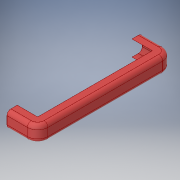
# Autodesk Inventor part: Bumper Fabric
Saved by Autodesk Inventor 2019.4 (Build 234330000, 330)
## iProperties
Created: 2020-01-22
Part Number: Bumper Fabric
Material: Fabric
Document SubType Name: Modeling
Designer: admin
Density: 0.9 g/cm^3
Appearance: Smooth - Red
Author: admin
Autodesk Inventor part; units mm, degrees
ref_plane "YZ Plane" through (0, 0, 0) normal (1, 0, 0) x (0, 1, 0)
ref_plane "XZ Plane" through (0, 0, 0) normal (0, 1, 0) x (-1, 0, 0)
ref_plane "XY Plane" through (0, 0, 0) normal (0, 0, 1) x (1, 0, 0)
sketch "Sketch1" plane through (0, 0, 0) normal (1, 0, 0) x (0, 1, 0)
  line L0 (0, 0) -> (0, 51.5)
  arc A0 (0, 51.5) -> (-31.5, 83) centre (-31.5, 51.5) ccw
  line L1 (-31.5, 83) -> (-95.5, 83)
  arc A1 (-95.5, 83) -> (-127, 51.5) centre (-95.5, 51.5) ccw
  line L2 (-127, 51.5) -> (-127, 0)
  line L3 (-127.5, 0) -> (-127.5, 51.5)
  arc A2 (-95.5, 83.5) -> (-127.5, 51.5) centre (-95.5, 51.5) ccw
  line L4 (-95.5, 83.5) -> (-31.5, 83.5)
  arc A3 (0.5, 51.5) -> (-31.5, 83.5) centre (-31.5, 51.5) ccw
  line L5 (0.5, 51.5) -> (0.5, 0)
  line L6 (0.5, 0) -> (0, 0)
  line L7 (-127, 0) -> (-127.5, 0)
  dimension "d0" = 31.5
  dimension "d1" = 31.5
  dimension "d2" = 51.5
  dimension "d3" = 127
  dimension "d4" = 51.5
  dimension "d5" = 0.5
  constraints: 16 end point, 8 point on circle, 4 centre point, 4 tangent, 2 horizontal, 2 vertical, 1 collinear, 4 other
  measures "d0" radius of A0
  measures "d1" radius of A1
  measures "d2" distance of L0.start L0.end
  measures "d3" distance between parallel lines of L2 L0
  measures "d4" distance of L2.start L2.end
  measures "d5" distance between parallel lines of L2 L3
extrude "Extrusion1" add sketch "Sketch1" along normal blind 165.1
sketch "Sketch2" plane through (165.1, 0, 0) normal (1, 0, 0) x (0, 0, -1)
  line L0 (-51.5, 0) -> (0, 0) projected
  line L1 (0, 0) -> (0, 0.5) projected
  line L2 (0, 0.5) -> (-51.5, 0.5) projected
  arc A0 (-51.5, 0.5) -> (-83.5, -31.5) centre (-51.5, -31.5) ccw projected
  line L3 (-83.5, -31.5) -> (-83.5, -95.5) projected
  arc A1 (-83.5, -95.5) -> (-51.5, -127.5) centre (-51.5, -95.5) ccw projected
  line L4 (-51.5, -127.5) -> (0, -127.5) projected
  line L5 (0, -127.5) -> (0, -127) projected
  line L6 (0, -127) -> (-51.5, -127) projected
  arc A2 (-83, -95.5) -> (-51.5, -127) centre (-51.5, -95.5) ccw projected
  line L7 (-83, -95.5) -> (-83, -31.5) projected
  arc A3 (-51.5, 0) -> (-83, -31.5) centre (-51.5, -31.5) ccw projected
  line L8 (-51.5, 0.5) -> (0, 0.5) projected
  line L9 (-20, 0.5) -> (-20, 0)
  line L10 (-51.5, 0) -> (0, 0) projected
  line L11 (-20, -127) -> (-20, -127.5)
  line L12 (0, -127.5) -> (-51.5, -127.5) projected
  dimension "d11" = 63
  constraints: 4 end point, 4 point on line, 2 collinear, 1 vertical
  measures "d11" distance between parallel lines of L7 L9
revolve "Revolution1" add sketch "Sketch2" angle 90 about axis through (165.1, 0, 0) along (0, 1, 0)
sketch "Sketch3" plane through (216.6, 0.5, 0) normal (0, 0, -1) x (-1, 0, 0)
  line L0 (216.6, 0) -> (216.6, -0.5) projected
  line L1 (216.6, 0) -> (0, 0) projected
  arc A0 (0, 0) -> (-32, -32) centre (0, -32) ccw projected
  line L2 (-32, -32) -> (-32, -96) projected
  arc A1 (-32, -96) -> (0, -128) centre (0, -96) ccw projected
  line L3 (216.6, -128) -> (0, -128) projected
  line L4 (216.6, -127.5) -> (216.6, -128) projected
  line L5 (216.6, -127.5) -> (0, -127.5) projected
  arc A2 (-31.5, -96) -> (0, -127.5) centre (0, -96) ccw projected
  line L6 (-31.5, -96) -> (-31.5, -32) projected
  arc A3 (0, -0.5) -> (-31.5, -32) centre (0, -32) ccw projected
  line L7 (216.6, -0.5) -> (0, -0.5) projected
  line L8 (216.6, -128) -> (51.5, -128) projected
  line L9 (51.5, -127.5) -> (51.5, -128)
  line L10 (216.6, -0.5) -> (51.5, -0.5) projected
  line L11 (216.6, 0) -> (51.5, 0) projected
  line L12 (51.5, -0.5) -> (51.5, 0)
  constraints: 4 end point, 1 perpendicular, 1 point on line, 1 vertical
extrude "Extrusion2" add sketch "Sketch3" along normal blind 930 contours L12 L7 A3 L6 A2 L5 L9 L3 A1 L2 A0 L1
ref_plane "Work Plane1" through (216.6, 0.5, -465) normal (0, 0, -1) x (-1, 0, 0)
mirror "Mirror1" about plane through (216.6, 0.5, -465) normal (0, 0, -1) of "Extrusion1", "Revolution1"
equation "\"d1\" = d0"
equation "\"d4\" = d2"
body "Solid1"
